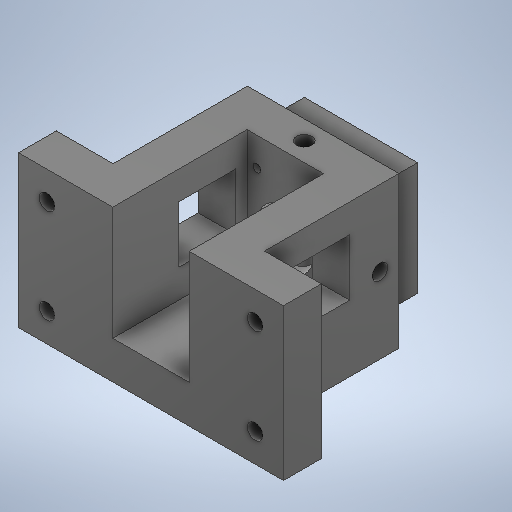
# Autodesk Inventor part: motor_bracket3
Saved by Autodesk Inventor 2026.2 (Build 302298010, 298A)
## iProperties
Created: 2026-04-13
Part Number: motor_bracket3
Material: ABS Plastic
Document SubType Name: Modeling
Designer: chris
Density: 1.06 g/cm^3
Appearance: Smooth - White
Author: chris
Autodesk Inventor part; units mm, degrees
ref_plane "YZ Plane" through (0, 0, 0) normal (1, 0, 0) x (0, 1, 0)
ref_plane "XZ Plane" through (0, 0, 0) normal (0, 1, 0) x (-1, 0, 0)
ref_plane "XY Plane" through (0, 0, 0) normal (0, 0, 1) x (1, 0, 0)
sketch "Sketch1" plane through (0, 0, 0) normal (0, 0, 1) x (1, 0, 0)
  line L0 (-20, -25.05) -> (20, -25.05)
  line L1 (20, -25.05) -> (20, 25.05)
  line L2 (20, 25.05) -> (-20, 25.05)
  line L3 (-20, 25.05) -> (-20, -25.05)
  line L4 (-20, -25.05) -> (20, 25.05) construction
  line L5 (20, -25.05) -> (-20, 25.05) construction
  point P0 (0, 0)
  dimension "d0" = 40
  dimension "d1" = 50.1
  constraints: 12 end point, 2 midpoint, 2 parallel, 1 horizontal, 1 perpendicular
  measures "d0" distance of L2.end L1.end
  measures "d1" distance of L1.end L0.end
extrude "Extrusion1" add sketch "Sketch1" against normal blind 45.5
sketch "Sketch2" plane through (0, 0, 0) normal (0, 0, 1) x (1, 0, 0)
  line L0 (-10.1, -15.05) -> (10.1, -15.05)
  line L1 (10.1, -15.05) -> (10.1, 25.05)
  line L2 (10.1, 25.05) -> (-10.1, 25.05)
  line L3 (-10.1, 25.05) -> (-10.1, -15.05)
  line L4 (-10.1, -15.05) -> (10.1, 25.05) construction
  line L5 (10.1, -15.05) -> (-10.1, 25.05) construction
  line L6 (20, 25.05) -> (-20, 25.05) projected
  point P0 (0, 0)
  point P1 (0, 5)
  dimension "d4" = 20.2
  dimension "d5" = 40.1
  constraints: 12 end point, 2 midpoint, 2 parallel, 1 collinear, 1 horizontal, 1 perpendicular
  measures "d4" distance of L2.end L1.end
  measures "d5" distance of L1.end L0.end
extrude "Extrusion2" cut sketch "Sketch2" against normal blind 35.5
sketch "Sketch3" plane through (0, 0, -35.5) normal (0, 0, 1) x (1, 0, 0)
  circle A0 centre (0, -5.05) radius 7.5
  line L0 (10.1, -15.05) -> (-10.1, -15.05) projected
  point P0 (0, 0)
  dimension "d8" = 15
  dimension "d9" = 10
  constraints: 1 centre point
  measures "d8" diameter of A0
  measures "d9" distance from line of L0 A0.centre
extrude "Extrusion3" cut sketch "Sketch3" against normal blind 6
sketch "Sketch4" plane through (0, 0, -45.5) normal (0, 0, -1) x (-1, 0, 0)
  line L0 (-14.95, -20) -> (14.95, -20)
  line L1 (14.95, -20) -> (14.95, 9.9)
  line L2 (14.95, 9.9) -> (-14.95, 9.9)
  line L3 (-14.95, 9.9) -> (-14.95, -20)
  line L4 (-14.95, -20) -> (14.95, 9.9) construction
  line L5 (14.95, -20) -> (-14.95, 9.9) construction
  line L6 (-20, -25.05) -> (20, -25.05) projected
  point P0 (0, 0)
  point P1 (0, -5.05)
  dimension "d12" = 29.9
  dimension "d13" = 29.9
  dimension "d14" = 20
  constraints: 12 end point, 2 midpoint, 2 parallel, 1 horizontal, 1 perpendicular
  measures "d12" distance of L2.end L1.end
  measures "d13" distance of L1.end L0.end
  measures "d14" distance from line of L6 point (0, -5.05)
extrude "Extrusion4" add sketch "Sketch4" along normal blind 10
sketch "Sketch5" plane through (20, -25.05, 0) normal (1, 0, 0) x (0, 0, -1)
  line L0 (17.5, 17.5) -> (32.5, 17.5)
  line L1 (32.5, 17.5) -> (32.5, 32.5)
  line L2 (32.5, 32.5) -> (17.5, 32.5)
  line L3 (17.5, 32.5) -> (17.5, 17.5)
  line L4 (17.5, 17.5) -> (32.5, 32.5) construction
  line L5 (32.5, 17.5) -> (17.5, 32.5) construction
  line L6 (45.5, 50.1) -> (45.5, 0) projected
  line L7 (0, 0) -> (45.5, 0) projected
  point P0 (0, 25.05)
  point P1 (25, 25)
  dimension "d17" = 15
  dimension "d18" = 15
  dimension "d19" = 13
  dimension "d20" = 17.5
  constraints: 12 end point, 2 midpoint, 2 parallel, 1 horizontal, 1 perpendicular
  measures "d17" distance of L2.end L1.end
  measures "d18" distance of L1.end L0.end
  measures "d19" distance between parallel lines of L6 L1
  measures "d20" distance between parallel lines of L7 L0
extrude "Extrusion5" cut sketch "Sketch5" against normal through all
sketch "Sketch6" plane through (-20, -25.05, 0) normal (0, -1, 0) x (1, 0, 0)
  line L0 (27.5, -17.5) -> (12.5, -17.5)
  line L1 (12.5, -17.5) -> (12.5, -32.5)
  line L2 (12.5, -32.5) -> (27.5, -32.5)
  line L3 (27.5, -32.5) -> (27.5, -17.5)
  line L4 (27.5, -17.5) -> (12.5, -32.5) construction
  line L5 (12.5, -17.5) -> (27.5, -32.5) construction
  line L6 (40, -45.5) -> (0, -45.5) projected
  point P0 (20, 0)
  point P1 (20, -25)
  dimension "d23" = 15
  dimension "d24" = 15
  dimension "d25" = 13
  constraints: 12 end point, 2 midpoint, 2 parallel, 1 horizontal, 1 perpendicular
  measures "d23" distance of L2.end L1.end
  measures "d24" distance of L1.end L0.end
  measures "d25" distance between parallel lines of L6 L2
extrude "Extrusion6" cut sketch "Sketch6" against normal through all
sketch "Sketch7" plane through (-20, 25.05, -45.5) normal (0, 1, 0) x (1, 0, 0)
  line L0 (0, -91) -> (40, -91)
  line L1 (40, -91) -> (40, 0)
  line L2 (40, 0) -> (0, 0)
  line L3 (0, 0) -> (0, -91)
  line L4 (0, -91) -> (40, 0) construction
  line L5 (40, -91) -> (0, 0) construction
  line L6 (0, 0) -> (40, 0) projected
  line L7 (40, -45.5) -> (40, 0) projected
  point P0 (20, -45.5)
  constraints: 12 end point, 2 collinear, 2 midpoint, 2 parallel, 1 horizontal, 1 perpendicular
extrude "Extrusion7" cut sketch "Sketch7" against normal blind 10.1
sketch "Sketch8" plane through (20, -25.05, 0) normal (1, 0, 0) x (0, 0, -1)
  line L0 (0, 0) -> (10, 0)
  line L1 (10, 0) -> (10, 40)
  line L2 (10, 40) -> (0, 40)
  line L3 (0, 40) -> (0, 0)
  line L4 (0, 0) -> (10, 40) construction
  line L5 (10, 0) -> (0, 40) construction
  line L6 (45.5, 40) -> (0, 40) projected
  line L7 (0, 0) -> (45.5, 0) projected
  line L8 (0, 0) -> (0, 40) projected
  point P0 (0, 25.05)
  point P1 (5, 20)
  dimension "d30" = 10
  constraints: 12 end point, 3 collinear, 2 midpoint, 2 parallel, 1 horizontal, 1 perpendicular
  measures "d30" distance of L0.start L0.end
extrude "Extrusion8" add sketch "Sketch8" along normal blind 15
mirror "Mirror1" about plane through (0, 0, 0) normal (1, 0, 0) of "Extrusion8"
sketch "Sketch9" plane through (0, 0, 0) normal (0, 0, 1) x (1, 0, 0)
  circle A0 centre (27.5, 7.45) radius 2.05
  circle A1 centre (27.5, -17.55) radius 2.05
  circle A2 centre (-27.5, 7.45) radius 2.05
  circle A3 centre (-27.5, -17.55) radius 2.05
  line L0 (35, 14.95) -> (10.1, 14.95) projected
  line L1 (35, 14.95) -> (35, -25.05) projected
  line L2 (-35, -25.05) -> (35, -25.05) projected
  line L3 (-35, 14.95) -> (-35, -25.05) projected
  line L4 (-10.1, 14.95) -> (-35, 14.95) projected
  point P0 (0, 0)
  dimension "d33" = 4.1
  dimension "d34" = 4.1
  dimension "d35" = 4.1
  dimension "d36" = 4.1
  dimension "d37" = 7.5
  dimension "d38" = 7.5
  dimension "d39" = 7.5
  dimension "d40" = 7.5
  dimension "d41" = 7.5
  dimension "d42" = 7.5
  dimension "d43" = 7.5
  dimension "d44" = 7.5
  constraints: 4 centre point
  measures "d33" diameter of A0
  measures "d34" diameter of A1
  measures "d35" diameter of A2
  measures "d36" diameter of A3
  measures "d37" distance from line of L0 A0.centre
  measures "d38" distance from line of L1 A0.centre
  measures "d39" distance from line of L1 A1.centre
  measures "d40" distance from line of L2 A1.centre
  measures "d41" distance from line of L2 A3.centre
  measures "d42" distance from line of L3 A3.centre
  measures "d43" distance from line of L3 A2.centre
  measures "d44" distance from line of L4 A2.centre
extrude "Extrusion9" cut sketch "Sketch9" against normal through all
sketch "Sketch10" plane through (20, -25.05, -10) normal (0, 0, -1) x (-1, 0, 0)
  circle A0 centre (-7.5, 32.5) radius 2.05 projected
  circle A1 centre (-7.5, 7.5) radius 2.05 projected
  circle A2 centre (47.5, 32.5) radius 2.05 projected
  circle A3 centre (47.5, 7.5) radius 2.05 projected
  circle A4 centre (-7.5, 32.5) radius 6
  circle A5 centre (47.5, 32.5) radius 6
  circle A6 centre (47.5, 7.5) radius 6
  circle A7 centre (-7.5, 7.5) radius 6
  point P0 (20, 25.05)
  dimension "d47" = 12
  dimension "d48" = 12
  dimension "d49" = 12
  dimension "d50" = 12
  constraints: 4 centre point, 4 coincident
  measures "d47" diameter of A4
  measures "d48" diameter of A5
  measures "d49" diameter of A6
  measures "d50" diameter of A7
extrude "Extrusion10" cut sketch "Sketch10" against normal blind 5
sketch "Sketch11" plane through (0, 0, -55.5) normal (0, 0, -1) x (-1, 0, 0)
  ellipse E0 centre (-7.952, -12.932) end of major axis (-8.818, -13.798) minor radius 1 (-9.07, -13.1556) -> (-8.1756, -14.05) ccw projected
  line L0 (8.1756, -14.05) -> (-8.1756, -14.05) projected
  ellipse E1 centre (7.952, -12.932) end of major axis (8.818, -13.798) minor radius 1 (8.1756, -14.05) -> (9.07, -13.1556) ccw projected
  line L1 (9.07, 23.1556) -> (9.07, -13.1556) projected
  ellipse E2 centre (7.952, 22.932) end of major axis (8.818, 23.798) minor radius 1 (9.07, 23.1556) -> (8.1756, 24.05) ccw projected
  line L2 (-8.1756, 24.05) -> (8.1756, 24.05) projected
  ellipse E3 centre (-7.952, 22.932) end of major axis (-8.818, 23.798) minor radius 1 (-8.1756, 24.05) -> (-9.07, 23.1556) ccw projected
  line L3 (-9.07, -13.1556) -> (-9.07, 23.1556) projected
  circle A0 centre (7.525, 22.55) radius 0.7835 projected
  circle A1 centre (-7.525, 22.55) radius 0.7835 projected
  circle A2 centre (7.525, 7.45) radius 0.7835 projected
  circle A3 centre (-7.525, 7.45) radius 0.7835 projected
  circle A4 centre (7.525, -12.55) radius 0.7835 projected
  circle A5 centre (-7.525, -12.55) radius 0.7835 projected
  circle A6 centre (0, -5.05) radius 6.4 projected
  point P0 (0, 0)
  constraints: 4 other
hole "Hole1" at (-7.525, 7.45, -55.5) at (-7.525, -12.55, -55.5) at (7.525, 7.45, -55.5) at (7.525, -12.55, -55.5) direction (0, 0, 1) diameter 2.1 end through all
sketch "Sketch12" plane through (0, 0, -55.5) normal (0, 0, -1) x (-1, 0, 0)
  circle A0 centre (7.525, 7.45) radius 1.05 projected
  circle A1 centre (7.525, -12.55) radius 1.05 projected
  circle A2 centre (-7.525, -12.55) radius 1.05 projected
  circle A3 centre (-7.525, 7.45) radius 1.05 projected
  circle A4 centre (7.525, 7.45) radius 2
  circle A5 centre (7.525, -12.55) radius 2
  circle A6 centre (-7.525, -12.55) radius 2
  circle A7 centre (-7.525, 7.45) radius 2
  point P0 (0, 0)
  dimension "d60" = 4
  dimension "d61" = 4
  dimension "d62" = 4
  dimension "d63" = 4
  constraints: 4 centre point, 4 coincident
  measures "d60" diameter of A4
  measures "d61" diameter of A5
  measures "d62" diameter of A6
  measures "d63" diameter of A7
extrude "Extrusion11" cut sketch "Sketch12" against normal blind 15 contours A0 | A1 | A2 | A3 | A4 | A5 | A6 | A7
sketch "Sketch13" plane through (20, -25.05, -45.5) normal (1, 0, 0) x (0, 0, -1)
  circle A0 centre (-5, 20) radius 2.05
  line L0 (-35.5, 0) -> (0, 0) projected
  line L1 (0, 40) -> (0, 0) projected
  point P0 (-45.5, 25.05)
  dimension "d66" = 4.1
  dimension "d67" = 20
  dimension "d68" = 5
  constraints: 1 centre point
  measures "d66" diameter of A0
  measures "d67" distance from line of L0 A0.centre
  measures "d68" distance from line of L1 A0.centre
extrude "Extrusion12" cut sketch "Sketch13" against normal through all
sketch "Sketch14" plane through (-20, 14.95, -45.5) normal (0, 1, 0) x (1, 0, 0)
  circle A0 centre (20, -5) radius 2.05
  line L0 (0, 0) -> (40, 0) projected
  point P0 (20, -45.5)
  dimension "d71" = 4.1
  dimension "d72" = 5
  constraints: 1 centre point
  measures "d71" diameter of A0
  measures "d72" distance from line of A0.centre L0
extrude "Extrusion13" cut sketch "Sketch14" against normal through all
body "Solid1"
